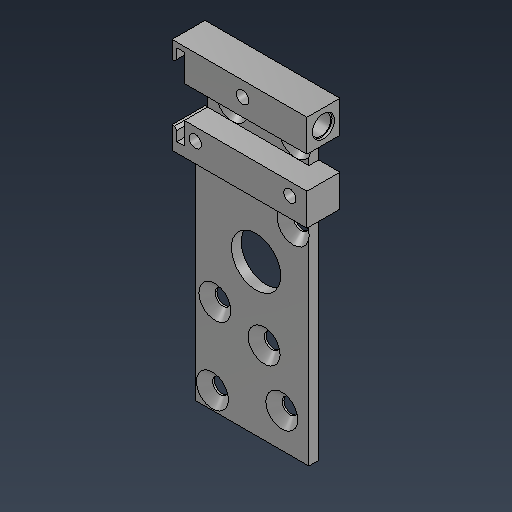
# Autodesk Inventor part: RightGearboxCover
Saved by Autodesk Inventor 2026.2 (Build 302298010, 298A)
## iProperties
Created: 2026-04-14
Part Number: RightGearboxCover
Material: Nylon 6/6
Document SubType Name: Modeling
Designer: szymo
Density: 1.13 g/cm^3
Appearance: Nylon 6(1)
Author: szymo
Autodesk Inventor part; units mm, degrees
ref_plane "YZ Plane" through (0, 0, 0) normal (1, 0, 0) x (0, 1, 0)
ref_plane "XZ Plane" through (0, 0, 0) normal (0, 1, 0) x (-1, 0, 0)
ref_plane "XY Plane" through (0, 0, 0) normal (0, 0, 1) x (1, 0, 0)
sketch "Sketch1" plane through (0, 0, 0) normal (0, 0, 1) x (1, 0, 0)
  circle A0 centre (14.7, -14.7) radius 14.7 construction
  circle A1 centre (14.7, -14.7) radius 4
  circle A2 centre (14.7, -14.7) radius 14 construction
  circle A3 centre (14.7, -55.6371) radius 14.7 construction
  line L0 (2.5, -17) -> (2.5, -1)
  line L1 (1.5, -17) -> (2.5, -17)
  line L2 (1.5, -1) -> (1.5, -17)
  line L3 (1.5, -1) -> (2.5, -1)
  circle A4 centre (12.35, -35.2722) radius 5
  circle A5 centre (9.2226, -23.0665) radius 1.25
  line L4 (27.4, 0) -> (0, 0)
  line L5 (0, 0) -> (0, -65.8371)
  line L6 (0, -65.8371) -> (23.1, -65.8371)
  line L7 (23.1, -65.8371) -> (23.1, -19.5)
  line L8 (23.1, -19.5) -> (27.4, -19.5)
  line L9 (27.4, -19.5) -> (27.4, -13)
  line L10 (27.4, -13) -> (23.1, -13)
  line L11 (23.1, -13) -> (23.1, -6.5)
  line L12 (23.1, -6.5) -> (27.4, -6.5)
  line L13 (27.4, -6.5) -> (27.4, 0)
  line L14 (23.1, -6.5) -> (9.1827, -6.5)
  line L15 (2.5, -1) -> (1, -1)
  line L16 (1, -1) -> (1, -3.5)
  line L17 (1, -3.5) -> (0, -3.5)
  line L18 (0, -15) -> (1, -15)
  line L19 (1, -15) -> (1, -17.5)
  line L20 (1, -17.5) -> (2.5, -17.5)
  line L21 (2.5, -17) -> (2.5, -17.5)
  line L22 (9.1827, -6.5) -> (2.5, -6.5)
  line L23 (23.1, -13) -> (2.5, -13)
  line L24 (23.1, -19.5) -> (0, -19.5)
  line L25 (23.1, -13) -> (23.1, -19.5)
  circle A6 centre (14.7, -55.6371) radius 14.7 projected
  circle A7 centre (14.7, -55.6371) radius 14 projected
  circle A8 centre (14.7, -14.7) radius 14.7 projected
  circle A9 centre (14.7, -14.7) radius 14 projected
  circle A10 centre (23.925, -15.5491) radius 0.75
  circle A11 centre (14.325, -3) radius 0.75
  circle A12 centre (4.725, -15.5491) radius 0.75
  circle A13 centre (9.2226, -23.0665) radius 1.25 projected
  arc A14 (5.455, -24.9226) -> (6.8523, -24.6489) centre (5.4549, -21.218) ccw projected
  arc A15 (6.8523, -24.6489) -> (7.0791, -24.9448) centre (9.2226, -23.0665) ccw projected
  arc A16 (7.0791, -24.9448) -> (6.4521, -26.2231) centre (10.0296, -27.1849) ccw projected
  arc A17 (6.4521, -26.2231) -> (6.8878, -26.5577) centre (9.2226, -23.0665) ccw projected
  arc A18 (6.8878, -26.5577) -> (7.9611, -25.6221) centre (5.0354, -23.3495) ccw projected
  arc A19 (7.9611, -25.6221) -> (8.3054, -25.7649) centre (9.2226, -23.0665) ccw projected
  arc A20 (8.3054, -25.7649) -> (8.4016, -27.1855) centre (11.9807, -26.2297) ccw projected
  arc A21 (8.4016, -27.1855) -> (8.9462, -27.2574) centre (9.2226, -23.0665) ccw projected
  arc A22 (8.9462, -27.2574) -> (9.4079, -25.9105) centre (5.7379, -25.4052) ccw projected
  arc A23 (9.4079, -25.9105) -> (9.7775, -25.862) centre (9.2226, -23.0665) ccw projected
  arc A24 (9.7775, -25.862) -> (10.5711, -27.0442) centre (13.1928, -24.4268) ccw projected
  arc A25 (10.5711, -27.0442) -> (11.0787, -26.8341) centre (9.2226, -23.0665) ccw projected
  arc A26 (11.0787, -26.8341) -> (10.805, -25.4368) centre (7.3742, -26.8342) ccw projected
  arc A27 (10.805, -25.4368) -> (11.1009, -25.21) centre (9.2226, -23.0665) ccw projected
  arc A28 (11.1009, -25.21) -> (12.3792, -25.837) centre (13.3411, -22.2595) ccw projected
  arc A29 (12.3792, -25.837) -> (12.7138, -25.4013) centre (9.2226, -23.0665) ccw projected
  arc A30 (12.7138, -25.4013) -> (11.7782, -24.3281) centre (9.5057, -27.2537) ccw projected
  arc A31 (11.7782, -24.3281) -> (11.921, -23.9837) centre (9.2226, -23.0665) ccw projected
  arc A32 (11.921, -23.9837) -> (13.3416, -23.8875) centre (12.3858, -20.3084) ccw projected
  arc A33 (13.3416, -23.8875) -> (13.4135, -23.3429) centre (9.2226, -23.0665) ccw projected
  arc A34 (13.4135, -23.3429) -> (12.0666, -22.8813) centre (11.5613, -26.5512) ccw projected
  arc A35 (12.0666, -22.8813) -> (12.0181, -22.5116) centre (9.2226, -23.0665) ccw projected
  arc A36 (12.0181, -22.5116) -> (13.2003, -21.7181) centre (10.583, -19.0963) ccw projected
  arc A37 (13.2003, -21.7181) -> (12.9902, -21.2104) centre (9.2226, -23.0665) ccw projected
  arc A38 (12.9902, -21.2104) -> (11.5929, -21.4841) centre (12.9904, -24.915) ccw projected
  arc A39 (11.5929, -21.4841) -> (11.3661, -21.1882) centre (9.2226, -23.0665) ccw projected
  arc A40 (11.3661, -21.1882) -> (11.9932, -19.9099) centre (8.4156, -18.9481) ccw projected
  arc A41 (11.9932, -19.9099) -> (11.5574, -19.5753) centre (9.2226, -23.0665) ccw projected
  arc A42 (11.5574, -19.5753) -> (10.4842, -20.5109) centre (13.4098, -22.7834) ccw projected
  arc A43 (10.4842, -20.5109) -> (10.1398, -20.3681) centre (9.2226, -23.0665) ccw projected
  arc A44 (10.1398, -20.3681) -> (10.0437, -18.9475) centre (6.4645, -19.9033) ccw projected
  arc A45 (10.0437, -18.9475) -> (9.499, -18.8756) centre (9.2226, -23.0665) ccw projected
  arc A46 (9.499, -18.8756) -> (9.0374, -20.2225) centre (12.7073, -20.7278) ccw projected
  arc A47 (9.0374, -20.2225) -> (8.6677, -20.271) centre (9.2226, -23.0665) ccw projected
  arc A48 (8.6677, -20.271) -> (7.8742, -19.0888) centre (5.2525, -21.7061) ccw projected
  arc A49 (7.8742, -19.0888) -> (7.3665, -19.2989) centre (9.2226, -23.0665) ccw projected
  arc A50 (7.3665, -19.2989) -> (7.6402, -20.6962) centre (11.0711, -19.2988) ccw projected
  arc A51 (7.6402, -20.6962) -> (7.3444, -20.923) centre (9.2226, -23.0665) ccw projected
  arc A52 (7.3444, -20.923) -> (6.066, -20.296) centre (5.1042, -23.8735) ccw projected
  arc A53 (6.066, -20.296) -> (5.7314, -20.7317) centre (9.2226, -23.0665) ccw projected
  arc A54 (5.7314, -20.7317) -> (6.667, -21.8049) centre (8.9396, -18.8793) ccw projected
  arc A55 (6.667, -21.8049) -> (6.5242, -22.1493) centre (9.2226, -23.0665) ccw projected
  arc A56 (6.5242, -22.1493) -> (5.1037, -22.2454) centre (6.0594, -25.8246) ccw projected
  arc A57 (5.1037, -22.2454) -> (5.0317, -22.7901) centre (9.2226, -23.0665) ccw projected
  arc A58 (5.0317, -22.7901) -> (6.3786, -23.2517) centre (6.8839, -19.5818) ccw projected
  arc A59 (6.3786, -23.2517) -> (6.4272, -23.6214) centre (9.2226, -23.0665) ccw projected
  arc A60 (6.4272, -23.6214) -> (5.245, -24.4149) centre (7.8623, -27.0367) ccw projected
  arc A61 (5.245, -24.4149) -> (5.455, -24.9226) centre (9.2226, -23.0665) ccw projected
  circle A62 centre (12.35, -35.2722) radius 5 projected
  circle A63 centre (12.35, -35.2722) radius 5.4 projected
  line L26 (1.5, -17) -> (1.5, -1) projected
  line L27 (2.5, -17) -> (1.5, -17) projected
  line L28 (2.5, -1) -> (2.5, -17) projected
  line L29 (2.5, -1) -> (1.5, -1) projected
  line L30 (27.4, -19.5) -> (27.4, -19.46)
  point P0 (4.1146, -65.8371)
  point P1 (0, -55.6371)
  point P2 (0.0031, -15)
  point P3 (0, -14.7)
  point P4 (26.4337, -19.5)
  point P5 (27.4, -19.5)
  point P6 (2.5, -6.4994)
  point P7 (1.5, -8.2308)
  point P8 (14.7, 0)
  point P9 (26.9004, -6.5)
  point P10 (23.1, -26.7636)
  dimension "d0" = 2
  dimension "d1" = 4.5
  dimension "d2" = 6.3
  dimension "d4" = 2.5
  dimension "d5" = 10
  dimension "d6" = 0.5
  dimension "d7" = 0.5
  dimension "d8" = 2.5
  dimension "d9" = 2.5
  dimension "d10" = 0.5
  dimension "d11" = 19.5
  dimension "d12" = 6.5
  dimension "d17" = 8
  dimension "d18" = 6.5
  dimension "d59" = 6.3
  constraints: 54 end point, 10 perpendicular, 9 centre point, 8 coincident, 8 collinear, 7 point on line, 7 vertical, 5 tangent, 4 horizontal, 2 parallel, 6 other
  measures "d0" distance edge to line of A0 L9
  measures "d1" distance edge to line of A3 L6
  measures "d2" distance edge to line of A0 L11
  measures "d4" diameter of A5
  measures "d5" diameter of A4
  measures "d6" distance between parallel lines of L1 L20
  measures "d7" distance between parallel lines of L2 L19
  measures "d8" distance between parallel lines of L20 L18
  measures "d9" distance between parallel lines of L17 L15
  measures "d10" distance between parallel lines of L16 L2
  measures "d11" distance between parallel lines of L4 L24
  measures "d12" distance between parallel lines of L24 L23
  measures "d17" diameter of A1
  measures "d18" distance between parallel lines of L4 L14
  measures "d59" distance edge to line of A0 L7
extrude "Extrusion1" add sketch "Sketch1" along normal blind 2 contours A1 L23 | A1 L23 L25 L24 A44 A45 A46 A48 A49 A50 A9 L18 L19 L20 L21 L0 | L23 A1 | A1 L23 L0 A9 L22 L14 L11 | L10 L9 L8 L25 | L14 L22 A9 L12 | L7 A9 A18 A19 A20 A21 A22 A23 A24 A25 A26 A27 A28 A29 A30 A31 A32 A33 A34 A35 A36 A37 A38 A39 A40 A41 A42 A43 A44 L24 | L0 L22 A9 | A9 L22 A8 L12 | L7 A8 L24 A9 A16 A17 A18 | A44 A43 A42 A41 A40 A39 A38 A37 A36 A35 A34 A33 A32 A31 A30 A29 A28 A27 A26 A25 A24 A23 A22 A21 A20 A19 A18 A9 A16 A15 A14 A61 A60 A59 A58 A57 A56 A55 A54 A53 A52 A51 A50 L24 A48 A47 A46 | L24 A46 A45 A44 | L0 L3 L15 L16 L17 L5 L4 A8 | A8 L4 L13 L12 | L7 A6 L5 L24 A8 | A18 A17 A16 A9 | A46 A47 A48 L24 | A9 L24 A8 L18 | L7 A7 L6 A6 | L24 L5 L18 A8 | A9 L24 A50 A51 A52 A53 A54 A55 A56 A57 A58 A59 A60 A61 A14 A15 A16 | L24 A50 A49 A48 | L7 L6 A7 | A6 L6 L5 | A5 | A10 | A11 | A12 | A63 picked at (0.53, -55.6401) picked at (11.9741, -51.5942)
ref_plane "Work Plane1" through (1, -19, 6.7) normal (0, 0, -1) x (0, 1, 0)
ref_plane "Work Plane2" through (1, -19, 6.7) normal (0, 0, -1) x (0, 1, 0)
extrude "Extrusion2" add sketch "Sketch1" along normal up to surface (6.7 mm away) contours A1 L23 | A1 L23 L25 L24 A44 A45 A46 A48 A49 A50 A9 L18 L19 L20 L21 L0 | L10 L9 L8 L25 | L14 L22 A9 L12 | A9 L22 A8 L12 | L24 A46 A45 A44 | L0 L3 L15 L16 L17 L5 L4 A8 | A8 L4 L13 L12 | A9 L24 A8 L18 | L24 L5 L18 A8 | L24 A50 A49 A48 | A10 | A11 | A12 picked at (13.7286, -14.48)
hole "Hole1" at (14.325, -3, 0) at (23.925, -15.5491, 0) at (4.725, -15.5491, 0) direction (0, 0, 1) diameter 2.5 end through all counterbore diameter 3 counterbore depth 0.5
extrude "Extrusion3" cut sketch "Sketch1" along normal blind 1.5 contours A1 L23 | L23 A1 | A5
chamfer "Chamfer1" distance 0.5 angle 45 2 edges at (1, -3.5, 3.35) (1, -15, 3.35)
sketch "Sketch2" plane through (0, 0, 2) normal (0, 0, 1) x (1, 0, 0)
  circle A0 centre (4, -46.5095) radius 3 projected
  circle A1 centre (3.5, -62.3371) radius 3 projected
  circle A2 centre (17.6, -58.8371) radius 3 projected
  circle A3 centre (14, -49.1746) radius 3 projected
  circle A4 centre (7.5, -9.75) radius 3 projected
  arc A5 (4.0542, -29.6883) -> (19.4959, -28.2768) centre (12.35, -35.2722) ccw projected
  arc A6 (9.7, -14.6801) -> (4.0542, -29.6883) centre (9.2226, -23.0665) ccw projected
  arc A7 (16.7181, -19.2746) -> (9.7, -14.6801) centre (14.7, -14.7) ccw projected
  arc A8 (17.618, -23.3446) -> (16.7181, -19.2746) centre (9.2226, -23.0665) ccw projected
  line L0 (27.4, 0) -> (27.4, -6.5) projected
  line L1 (0, 0) -> (27.4, 0) projected
  line L2 (0, -3.5) -> (0, 0) projected
  line L3 (1, -3.5) -> (0, -3.5) projected
  line L4 (1, -1) -> (1, -3.5) projected
  line L5 (2.5, -1) -> (1, -1) projected
  line L6 (2.5, -17.5) -> (2.5, -1) projected
  line L7 (1, -17.5) -> (2.5, -17.5) projected
  line L8 (1, -15) -> (1, -17.5) projected
  line L9 (0, -15) -> (1, -15) projected
  line L10 (0, -65.8371) -> (0, -15) projected
  line L11 (13.0938, -65.8371) -> (8.9062, -65.8371) projected
  line L12 (23.1, -6.5) -> (23.1, -65.8371) projected
  line L13 (27.4, -6.5) -> (23.1, -6.5) projected
  arc A9 (15.0114, -33.8876) -> (14.5438, -37.3185) centre (12.35, -35.2722) ccw projected
  line L14 (15.0114, -33.8876) -> (14.5438, -37.3185) projected
  circle A10 centre (20.3345, -9.75) radius 2.25 projected
  arc A11 (19.4959, -28.2768) -> (17.618, -23.3446) centre (19.8907, -25.3029) ccw projected
  line L15 (6.0938, -65.8371) -> (6.0938, -65.3371) projected
  line L16 (6.0938, -65.3371) -> (8.9062, -65.3371) projected
  line L17 (8.9062, -65.3371) -> (8.9062, -65.8371) projected
  line L18 (13.0938, -65.8371) -> (13.0938, -65.3371) projected
  line L19 (13.0938, -65.3371) -> (15.9062, -65.3371) projected
  line L20 (15.9062, -65.3371) -> (15.9062, -65.8371) projected
  line L21 (23.1, -65.8371) -> (15.9062, -65.8371) projected
  line L22 (6.0938, -65.8371) -> (0, -65.8371) projected
  point P0 (23.1, -24.1891)
  point P1 (12.35, -35.2722)
  constraints: 1 coincident
hole "Hole4" at (7.5, -9.75, 2) at (20.3345, -9.75, 2) at (19.8907, -25.3029, 2) at (14, -49.1746, 2) at (17.6, -58.8371, 2) at (3.5, -62.3371, 2) at (4, -46.5095, 2) direction (0, 0, -1) diameter 3.2 depth 5 countersink diameter 6.5 countersink angle 90 clearance for "Countersunk Flat Head Screw ISO 2009/7046" size "M3" standard "ISO"
sketch "Sketch3" plane through (27.4, -6.5, 0) normal (1, 0, 0) x (0, 0, -1)
  line L0 (0, 0) -> (0, 6.5) projected
  line L1 (0, 6.5) -> (-6.7, 6.5) projected
  line L2 (-6.7, 0) -> (-6.7, 6.5) projected
  line L3 (0, 0) -> (-6.7, 0) projected
  line L4 (0, 0) -> (-6.7, 0) projected
  line L5 (0, 6.5) -> (-6.7, 0)
  line L6 (-6.7, 6.5) -> (0, 0)
  point P0 (0, 6.5)
  point P1 (-3.35, 3.25)
  constraints: 4 end point, 2 midpoint
hole "Hole5" at (27.4, -3.25, 3.35) direction (-1, 0, 0) diameter 4 depth 6.5 counterbore diameter 4.5 counterbore depth 0.5
body "Solid1"
